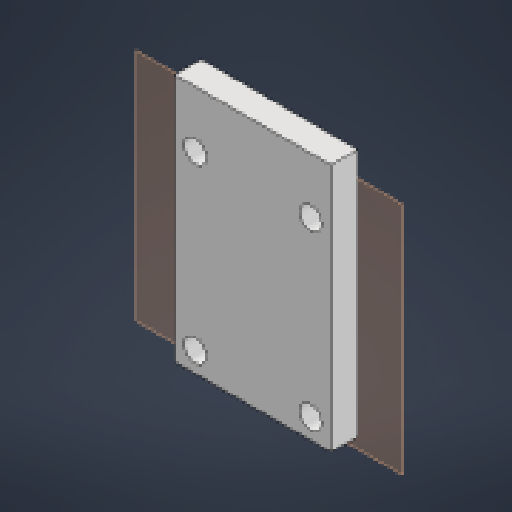
# Autodesk Inventor part: KickerMount_R
Saved by Autodesk Inventor 2024.2 (Build 282272000, 272)
## iProperties
Created: 2023-12-22
Part Number: KickerMount_R
Material: 一般
Document SubType Name: Modeling
Designer: Hanaoka
Density: 1 g/cm^3
Appearance: 既定
Author: Hanaoka
Autodesk Inventor part; units mm, degrees
ref_plane "YZ Plane" through (0, 0, 0) normal (1, 0, 0) x (0, 1, 0)
ref_plane "XZ Plane" through (0, 0, 0) normal (0, 1, 0) x (-1, 0, 0)
ref_plane "XY Plane" through (0, 0, 0) normal (0, 0, 1) x (1, 0, 0)
ref_plane "作業平面1" through (0, 0, 0) normal (0, 0, 1) x (1, 0, 0)
sketch "スケッチ1" plane through (0, 0, 0) normal (0, 0, 1) x (1, 0, 0)
  circle A0 centre (-6, -21.7) radius 1.25 projected
  circle A1 centre (-19, -21.7) radius 1.25 projected
  circle A2 centre (-19, -2.3) radius 1.25 projected
  circle A3 centre (-6, -2.3) radius 1.25 projected
  line L0 (0, -24) -> (-27.3, -24) projected
  line L1 (-3.7, -24) -> (-3.7, 4)
  line L2 (-3.7, 4) -> (-21.3, 4)
  line L3 (-21.3, 4) -> (-21.3, -24)
  circle A4 centre (-6, -21.7) radius 2.3 construction
  circle A5 centre (-19, -21.7) radius 2.3 construction
  point P0 (0, 0)
  dimension "d0" = 28
  constraints: 6 end point, 3 tangent, 2 centre point, 2 coincident, 2 point on line, 2 vertical, 1 equal radius, 1 horizontal
  measures "d0" distance of L1.start L1.end
extrude "押し出し1" add sketch "スケッチ1" along normal blind 3
